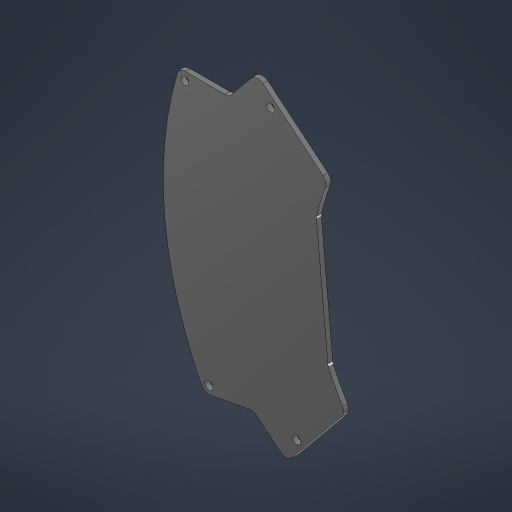
# Autodesk Inventor part: MainMCU_PCB
Saved by Autodesk Inventor 2024.2 (Build 282272000, 272)
## iProperties
Created: 2023-12-21
Part Number: MainMCU_PCB
Material: 一般
Document SubType Name: Modeling
Designer: Hanaoka
Density: 1 g/cm^3
Appearance: 既定
Author: Hanaoka
Autodesk Inventor part; units mm, degrees
ref_plane "YZ Plane" through (0, 0, 0) normal (1, 0, 0) x (0, 1, 0)
ref_plane "XZ Plane" through (0, 0, 0) normal (0, 1, 0) x (-1, 0, 0)
ref_plane "XY Plane" through (0, 0, 0) normal (0, 0, 1) x (1, 0, 0)
sketch "スケッチ1" plane through (0, 0, 0) normal (0, 0, 1) x (1, 0, 0)
  circle A0 centre (21.0053, 4.8422) radius 2 projected
  circle A1 centre (0, 0) radius 2 projected
  circle A2 centre (81.1718, -23.4817) radius 63 projected
  arc A3 (-1.9212, 0.5558) -> (4.0884, -62.7297) centre (81.1718, -23.4817) ccw
  line L0 (0, 2) -> (9.827, 2)
  line L1 (11.3686, 2.7258) -> (16.3193, 8.7154)
  line L2 (19.135, 8.9828) -> (33.9243, -3.2413)
  line L3 (8.2062, 4.3935) -> (1.7773, 9.7074) projected
  line L4 (40.3283, 40.1171) -> (11.022, 4.6609) projected
  arc A4 (9.827, 2) -> (11.3686, 2.7258) centre (9.827, 4) ccw
  arc A5 (19.135, 8.9828) -> (16.3193, 8.7154) centre (17.8609, 7.4412) ccw
  arc A6 (34.5163, -5.502) -> (38.7345, -49.9217) centre (81.1718, -23.4817) ccw
  circle A7 centre (5.8707, -61.8222) radius 2 projected
  circle A8 centre (27.412, -62.6241) radius 2 projected
  line L5 (81.1718, -23.4817) -> (18.1718, -23.4817) construction
  line L6 (38.5786, -52.2535) -> (26.3545, -67.0427)
  line L7 (17.573, -64.3252) -> (53.0292, -93.6315) projected
  line L8 (17.573, -64.3252) -> (53.0292, -93.6315) projected
  line L9 (9.4434, -71.0215) -> (14.7573, -64.5926) projected
  line L10 (23.5388, -67.3101) -> (17.5492, -62.3594)
  arc A9 (23.5388, -67.3101) -> (26.3545, -67.0427) centre (24.813, -65.7685) ccw
  line L11 (15.8985, -61.9368) -> (6.2472, -63.7865)
  arc A10 (17.5492, -62.3594) -> (15.8985, -61.9368) centre (16.275, -63.901) ccw
  arc A11 (34.5163, -5.502) -> (33.9243, -3.2413) centre (32.6501, -4.7828) ccw
  arc A12 (38.5786, -52.2535) -> (38.7345, -49.9217) centre (37.037, -50.9793) ccw
  circle A13 centre (5.8707, -61.8222) radius 1
  circle A14 centre (27.412, -62.6241) radius 1
  circle A15 centre (21.0053, 4.8422) radius 1
  circle A16 centre (0, 0) radius 1
  line L12 (0, 0) -> (5.8707, -61.8222) construction
  line L13 (32.2852, -12.9887) -> (35.1341, -42.9887)
  point P0 (0, 0)
  point P1 (35.0508, -4.1723)
  point P2 (39.5096, -51.127)
  dimension "d0" = 1.5
  dimension "d1" = 2
  dimension "d3" = 50
  dimension "d8" = 2
  dimension "d9" = 2
  dimension "d12" = 30
  constraints: 24 point on circle, 18 end point, 17 tangent, 12 centre point, 7 equal radius, 6 coincident, 4 parallel, 3 perpendicular, 2 horizontal, 2 point on line, 1 horizontal alignment, 1 other
  measures "d0" distance between parallel lines of L1 L4
  measures "d1" radius of A4
  measures "d3" radius of A6
  measures "d8" radius of A11
  measures "d9" diameter of A13
  measures "d12" vertical distance of L13.start L13.end
extrude "押し出し1" add sketch "スケッチ1" along normal blind 1.2 contours A0 | A8 | L2 A2 L6 A9 L10 A10 L11 A7 A3 A1 L0 A4 L1 A5 | L2 A11 A6 A12 L6 A2 | L13 A6 | A1 | A7
fillet "フィレット1" radius 2 2 edges at (35.1341, -42.9887, 0.6) (32.2852, -12.9887, 0.6)
